Autodesk Inventor part; units mm, degrees
(part 2 of 4)
  line L378 (5.5115, 49.3393) -> (5.5188, 49.3267)
  arc A125 (6.0858, 49.2107) -> (6.0188, 49.4607) centre (5.5858, 49.2107) ccw
  arc A126 (5.4445, 49.5893) -> (5.5115, 49.3393) centre (5.9445, 49.5893) ccw
  arc A127 (5.9445, 49.7233) -> (6.0115, 49.4733) centre (6.4445, 49.7233) ccw
  arc A128 (4.8374, 49.2618) -> (4.7704, 49.5118) centre (4.3374, 49.2618) ccw
  line L379 (4.2751, 50.3697) -> (4.7704, 49.5118)
  line L380 (4.8128, 49.4383) -> (3.7356, 50.3041) construction
  line L381 (6.0188, 49.4607) -> (6.0115, 49.4733)
  arc A129 (2.9678, 49.0767) -> (2.9008, 49.3267) centre (2.4678, 49.0767) ccw
  arc A130 (3.4678, 49.2107) -> (3.4008, 49.4607) centre (2.9678, 49.2107) ccw
  arc A131 (6.0858, 42.4055) -> (6.1549, 42.1519) centre (6.5858, 42.4055) ccw
  line L382 (6.0858, 42.4055) -> (6.0858, 49.2107)
  line L383 (5.5858, 49.0767) -> (5.5858, 42.2693)
  line L384 (6.0858, 49.2776) -> (5.5858, 42.2012) construction
  line L385 (6.0858, 42.2012) -> (5.5858, 49.2776) construction
  arc A132 (5.5858, 42.2693) -> (5.6549, 42.0157) centre (6.0858, 42.2693) ccw
  line L386 (6.0513, 42.328) -> (9.5345, 35.4232) construction
  line L387 (5.6549, 42.0157) -> (9.4309, 35.5993)
  line L388 (9.9655, 35.6768) -> (5.6203, 42.0744) construction
  line L389 (9.9309, 35.7355) -> (6.1549, 42.1519)
  arc A133 (9.5, 35.3457) -> (9.4309, 35.5993) centre (9, 35.3457) ccw
  arc A134 (10, 35.4819) -> (9.9309, 35.7355) centre (9.5, 35.4819) ccw
  line L390 (9.5, 35.3457) -> (9.5, 34.85)
  line L391 (9.5, 34.85) -> (8.35, 34.85)
  line L392 (8.35, 34.85) -> (8.35, 34.05)
  line L393 (10, 34.85) -> (9.5, 35.55) construction
  line L394 (10, 35.55) -> (9.5, 34.85) construction
  line L395 (10, 34.85) -> (10, 35.4819)
  line L396 (8.35, 34.05) -> (11.15, 34.05)
  line L397 (9.5, 34.85) -> (10, 34.85)
  line L398 (11.15, 34.85) -> (10, 34.85)
  line L399 (11.15, 34.05) -> (11.15, 34.85)
  line L400 (8.35, 14.55) -> (11.15, 14.55)
  line L401 (8.35, 15.35) -> (8.35, 14.55)
  line L402 (9.5, 15.35) -> (8.35, 15.35)
  line L403 (9.5, 15.35) -> (10, 15.35)
  line L404 (11.15, 14.55) -> (11.15, 15.35)
  line L405 (11.15, 15.35) -> (10, 15.35)
  line L406 (9.5, 15.8491) -> (9.5, 15.35)
  line L407 (10, 15.35) -> (10, 15.983)
  line L408 (9.75, 15.35) -> (9.75, 16.05)
  line L409 (10, 15.35) -> (9.5, 16.05) construction
  line L410 (10, 16.05) -> (9.5, 15.35) construction
  line L411 (10, 16.05) -> (9.5, 16.05)
  arc A135 (9.5, 15.8491) -> (9.4331, 16.099) centre (9, 15.8491) ccw
  line L412 (9.5335, 15.9251) -> (9.9665, 16.1749)
  arc A136 (10, 15.983) -> (9.9331, 16.2329) centre (9.5, 15.983) ccw
  arc A137 (10, -3.517) -> (9.933, -3.267) centre (9.5, -3.517) ccw
  line L413 (9.5335, -3.575) -> (9.9665, -3.325)
  line L414 (9.933, -3.267) -> (3.5348, 7.8151)
  line L415 (9.9665, -3.325) -> (3.0013, 7.7391) construction
  line L416 (3.0348, 7.6811) -> (9.433, -3.401)
  line L417 (3.4343, 7.9891) -> (9.5335, -3.575) construction
  arc A138 (3.4678, 8.0651) -> (3.5348, 7.8151) centre (3.9678, 8.0651) ccw
  arc A139 (2.9678, 7.9311) -> (3.0348, 7.6811) centre (3.4678, 7.9311) ccw
  arc A140 (9.5, -3.651) -> (9.433, -3.401) centre (9, -3.651) ccw
  line L418 (10, -3.45) -> (9.5, -3.45)
  line L419 (9.5, -3.651) -> (9.5, -4.15)
  line L420 (10, -4.15) -> (10, -3.517)
  line L421 (9.5, -4.15) -> (8.35, -4.15)
  line L422 (9.5, -4.15) -> (10, -4.15)
  line L423 (11.15, -4.15) -> (10, -4.15)
  line L424 (8.35, -4.15) -> (8.35, -4.95)
  line L425 (8.35, -4.95) -> (11.15, -4.95)
  line L426 (11.15, -4.95) -> (11.15, -4.15)
  arc A141 (2.1588, -9.1677) -> (2.2258, -9.4177) centre (2.6588, -9.1677) ccw
  arc A142 (1.6588, -9.3016) -> (1.7258, -9.5516) centre (2.1588, -9.3016) ccw
  line L427 (0.3498, -26.5344) -> (0.3498, 49.0767)
  line L428 (0.8498, 49.2107) -> (0.8498, -26.4004)
  line L429 (1.6588, 49.0767) -> (1.6588, -9.3016)
  line L430 (2.1588, 49.2776) -> (1.6588, -9.3686) construction
  line L431 (2.1588, -9.3686) -> (1.6588, 49.2776) construction
  line L432 (2.1588, -9.1677) -> (2.1588, 49.2107)
  line L433 (2.9678, 7.9311) -> (2.9678, 49.0767)
  line L434 (3.4678, 7.8641) -> (2.9678, 49.2776) construction
  line L435 (3.4678, 49.2776) -> (2.9678, 7.8641) construction
  line L436 (3.4678, 49.2107) -> (3.4678, 8.0651)
  line L437 (4.3374, 49.1278) -> (4.3374, 25.0639)
  line L438 (4.8374, 25.1978) -> (4.8374, 49.2618)
  line L439 (4.8374, 49.3098) -> (4.3374, 25.002) construction
  line L440 (4.8374, 25.002) -> (4.3374, 49.3098) construction
  line L441 (9.5335, -23.075) -> (9.9665, -22.825)
  line L442 (1.7258, -9.5516) -> (9.433, -22.901)
  line L443 (2.1253, -9.2436) -> (9.5335, -23.075) construction
  line L444 (9.9665, -22.825) -> (1.6923, -9.4936) construction
  line L445 (2.1253, -9.2436) -> (1.6923, -9.4936)
  line L446 (9.933, -22.767) -> (2.2258, -9.4177)
  line L447 (9.5, -23.65) -> (10, -23.65)
  line L448 (9.5, -23.151) -> (9.5, -23.65)
  line L449 (10, -23.65) -> (10, -23.017)
  line L450 (10, -23.65) -> (9.5, -22.95) construction
  line L451 (10, -22.95) -> (9.5, -22.95)
  line L452 (10, -22.95) -> (9.5, -23.65) construction
  arc A143 (9.5, -23.151) -> (9.433, -22.901) centre (9, -23.151) ccw
  line L453 (8.35, -24.45) -> (11.15, -24.45)
  arc A144 (10, -23.017) -> (9.933, -22.767) centre (9.5, -23.017) ccw
  line L454 (11.15, -23.65) -> (10, -23.65)
  line L455 (11.15, -24.45) -> (11.15, -23.65)
  arc A145 (0.8498, -26.4004) -> (0.9168, -26.6504) centre (1.3498, -26.4004) ccw
  line L456 (9.5, -23.65) -> (8.35, -23.65)
  line L457 (8.35, -23.65) -> (8.35, -24.45)
  line L458 (9.933, -42.267) -> (0.9168, -26.6504)
  line L459 (9.9665, -42.325) -> (0.3833, -26.7264) construction
  line L460 (0.8163, -26.4764) -> (9.5335, -42.575) construction
  line L461 (0.4168, -26.7844) -> (9.433, -42.401)
  arc A146 (0.3498, -26.5344) -> (0.4168, -26.7844) centre (0.8498, -26.5344) ccw
  line L462 (0.8163, -26.4764) -> (0.3833, -26.7264)
  line L463 (9.75, -48.75) -> (9.75, -43.95)
  line L464 (11.15, -43.95) -> (8.35, -43.95)
  line L465 (11.15, -43.15) -> (11.15, -43.95)
  arc A147 (9.5, -42.651) -> (9.433, -42.401) centre (9, -42.651) ccw
  arc A148 (10, -42.517) -> (9.933, -42.267) centre (9.5, -42.517) ccw
  line L466 (9.5, -42.651) -> (9.5, -43.15)
  line L467 (8.35, -43.15) -> (9.5, -43.15)
  line L468 (8.35, -43.95) -> (8.35, -43.15)
  line L469 (10, -43.15) -> (10, -42.517)
  line L470 (10, -42.45) -> (9.5, -43.15) construction
  line L471 (9.5, -43.15) -> (10, -43.15)
  line L472 (10, -43.15) -> (11.15, -43.15)
  line L473 (10, -43.15) -> (9.5, -42.45) construction
  line L474 (9.9331, 16.2329) -> (4.9043, 24.9479)
  line L475 (9.9665, 16.1749) -> (4.3679, 24.8771) construction
  line L476 (4.801, 25.127) -> (9.5335, 15.9251) construction
  line L477 (4.4043, 24.814) -> (9.4331, 16.099)
  arc A149 (4.8374, 25.1978) -> (4.9043, 24.9479) centre (5.3374, 25.1978) ccw
  arc A150 (4.3374, 25.0639) -> (4.4043, 24.814) centre (4.8374, 25.0639) ccw
  line L478 (-11.15, 54.35) -> (-11.15, 53.55)
  line L479 (-10.0555, 54.35) -> (-11.15, 54.35)
  line L480 (-11.15, 53.55) -> (-8.35, 53.55)
  line L481 (-8.35, 54.35) -> (-9.5705, 54.35)
  line L482 (-8.35, 53.55) -> (-8.35, 54.35)
  line L483 (-10.0555, 54.35) -> (-10.0555, 60.0191)
  line L484 (-10.0555, 60.0191) -> (-9.5705, 60.0191)
  line L485 (-9.5705, 60.0191) -> (-9.5705, 54.35)
  line L486 (-9.5705, 60.0191) -> (-10.0168, 54.35) construction
  line L487 (-9.5705, 54.2285) -> (-10.0555, 60.0191) construction
  line L488 (-9.5705, 54.35) -> (-10.0555, 54.35)
  circle A151 centre (-9.8055, 60.0191) radius 0.75
  line L489 (-22.0555, 60.0187) -> (-21.5555, 60.0187)
  circle A152 centre (-21.8055, 60.0191) radius 0.75
  line L490 (-17.5555, 60.0191) -> (-18.0555, 60.0191)
  circle A153 centre (-17.8055, 60.0191) radius 0.75
  line L491 (-13.5555, 60.0191) -> (-14.0555, 60.0191)
  circle A154 centre (-13.8055, 60.0191) radius 0.75
  arc A155 (-19.2919, 52.8573) -> (-19.2249, 52.6073) centre (-18.7919, 52.8573) ccw
  arc A156 (-19.7919, 52.7233) -> (-19.7249, 52.4733) centre (-19.2919, 52.7233) ccw
  line L492 (-19.2919, 55.5191) -> (-19.2919, 52.8573)
  line L493 (-19.2919, 55.5191) -> (-19.7919, 52.6564) construction
  line L494 (-19.2919, 52.6564) -> (-19.7919, 55.5191) construction
  line L495 (-19.7919, 55.5191) -> (-19.2919, 55.5191)
  circle A157 centre (-19.5419, 55.5191) radius 0.75
  line L496 (-17.5555, 60.0191) -> (-18.0555, 51.916) construction
  line L497 (-17.5555, 51.916) -> (-18.0555, 60.0191) construction
  line L498 (-17.5555, 52.117) -> (-17.5555, 60.0191)
  line L499 (-18.0555, 60.0191) -> (-18.0555, 51.983)
  line L500 (-21.5555, 60.0187) -> (-21.5555, 54.5107)
  line L501 (-21.5555, 60.0187) -> (-22.0555, 54.3101) construction
  line L502 (-21.5555, 54.3101) -> (-22.0555, 60.0187) construction
  line L503 (-22.0555, 54.3767) -> (-22.0555, 60.0187)
  line L504 (-19.7919, 52.7233) -> (-19.7919, 55.5191)
  line L505 (-15.7919, 55.5191) -> (-15.2919, 55.5191)
  circle A158 centre (-15.5419, 55.5191) radius 0.75
  line L506 (-13.5555, 49.7233) -> (-13.5555, 60.0191)
  line L507 (-14.0555, 60.0191) -> (-13.5555, 49.5223) construction
  line L508 (-14.0555, 49.5223) -> (-13.5555, 60.0191) construction
  line L509 (-14.0555, 60.0191) -> (-14.0555, 49.5893)
  line L510 (-15.2919, 55.5191) -> (-15.2919, 50.6197)
  line L511 (-15.7919, 50.4857) -> (-15.7919, 55.5191)
  line L512 (-15.2919, 55.5191) -> (-15.7919, 50.4326) construction
  line L513 (-15.2919, 50.4326) -> (-15.7919, 55.5191) construction
  arc A159 (-15.7919, 50.4857) -> (-15.7249, 50.2357) centre (-15.2919, 50.4857) ccw
  arc A160 (-15.2919, 50.6197) -> (-15.2249, 50.3697) centre (-14.7919, 50.6197) ccw
  arc A161 (-21.5555, 54.5107) -> (-21.4885, 54.2607) centre (-21.0555, 54.5107) ccw
  arc A162 (-22.0555, 54.3767) -> (-21.9885, 54.1267) centre (-21.5555, 54.3767) ccw
  arc A163 (-19.1502, 49.0767) -> (-19.2172, 49.3267) centre (-19.6502, 49.0767) ccw
  line L514 (-21.589, 54.4347) -> (-19.1167, 49.1526) construction
  line L515 (-21.4885, 54.2607) -> (-18.7172, 49.4607)
  line L516 (-19.2172, 49.3267) -> (-21.9885, 54.1267)
  line L517 (-18.6837, 49.4026) -> (-22.022, 54.1847) construction
  arc A164 (-17.3412, 49.2107) -> (-17.4082, 49.4607) centre (-17.8412, 49.2107) ccw
  arc A165 (-17.8412, 49.0767) -> (-17.9082, 49.3267) centre (-18.3412, 49.0767) ccw
  arc A166 (-18.6502, 49.2107) -> (-18.7172, 49.4607) centre (-19.1502, 49.2107) ccw
  line L518 (-16.0992, 49.4607) -> (-17.4885, 51.867)
  line L519 (-16.0657, 49.4026) -> (-18.022, 51.791) construction
  line L520 (-17.589, 52.041) -> (-16.4987, 49.1526) construction
  line L521 (-17.9885, 51.733) -> (-16.5992, 49.3267)
  line L522 (-19.3254, 52.7814) -> (-17.8077, 49.1526) construction
  line L523 (-19.2249, 52.6073) -> (-17.4082, 49.4607)
  line L524 (-17.9082, 49.3267) -> (-19.7249, 52.4733)
  line L525 (-17.3747, 49.4026) -> (-19.7584, 52.5314) construction
  arc A167 (-17.5555, 52.117) -> (-17.4885, 51.867) centre (-17.0555, 52.117) ccw
  arc A168 (-18.0555, 51.983) -> (-17.9885, 51.733) centre (-17.5555, 51.983) ccw
  line L526 (-15.2296, 49.3778) -> (-15.7249, 50.2357)
  line L527 (-15.3314, 50.5541) -> (-15.1202, 49.1883) construction
  arc A169 (-15.1626, 49.1278) -> (-15.2296, 49.3778) centre (-15.6626, 49.1278) ccw
  arc A170 (-13.9142, 49.0767) -> (-13.9812, 49.3267) centre (-14.4142, 49.0767) ccw
  line L528 (-13.9885, 49.3393) -> (-13.9812, 49.3267)
  arc A171 (-13.4142, 49.2107) -> (-13.4812, 49.4607) centre (-13.9142, 49.2107) ccw
  arc A172 (-14.0555, 49.5893) -> (-13.9885, 49.3393) centre (-13.5555, 49.5893) ccw
  arc A173 (-13.5555, 49.7233) -> (-13.4885, 49.4733) centre (-13.0555, 49.7233) ccw
  arc A174 (-14.6626, 49.2618) -> (-14.7296, 49.5118) centre (-15.1626, 49.2618) ccw
  line L529 (-15.2249, 50.3697) -> (-14.7296, 49.5118)
  line L530 (-14.6872, 49.4383) -> (-15.7644, 50.3041) construction
  line L531 (-13.4812, 49.4607) -> (-13.4885, 49.4733)
  arc A175 (-16.5322, 49.0767) -> (-16.5992, 49.3267) centre (-17.0322, 49.0767) ccw
  arc A176 (-16.0322, 49.2107) -> (-16.0992, 49.4607) centre (-16.5322, 49.2107) ccw
  arc A177 (-13.4142, 42.4055) -> (-13.3451, 42.1519) centre (-12.9142, 42.4055) ccw
  line L532 (-13.4142, 42.4055) -> (-13.4142, 49.2107)
  line L533 (-13.9142, 49.0767) -> (-13.9142, 42.2693)
  line L534 (-13.4142, 49.2776) -> (-13.9142, 42.2012) construction
  line L535 (-13.4142, 42.2012) -> (-13.9142, 49.2776) construction
  arc A178 (-13.9142, 42.2693) -> (-13.8451, 42.0157) centre (-13.4142, 42.2693) ccw
  line L536 (-13.4487, 42.328) -> (-9.9655, 35.4232) construction
  line L537 (-13.8451, 42.0157) -> (-10.0691, 35.5993)
  line L538 (-9.5345, 35.6768) -> (-13.8797, 42.0744) construction
  line L539 (-9.5691, 35.7355) -> (-13.3451, 42.1519)
  arc A179 (-10, 35.3457) -> (-10.0691, 35.5993) centre (-10.5, 35.3457) ccw
  arc A180 (-9.5, 35.4819) -> (-9.5691, 35.7355) centre (-10, 35.4819) ccw
  line L540 (-10, 35.3457) -> (-10, 34.85)
  line L541 (-10, 34.85) -> (-11.15, 34.85)
  line L542 (-11.15, 34.85) -> (-11.15, 34.05)
  line L543 (-9.5, 34.85) -> (-10, 35.55) construction
  line L544 (-9.5, 35.55) -> (-10, 34.85) construction
  line L545 (-9.5, 34.85) -> (-9.5, 35.4819)
  line L546 (-11.15, 34.05) -> (-8.35, 34.05)
  line L547 (-10, 34.85) -> (-9.5, 34.85)
  line L548 (-8.35, 34.85) -> (-9.5, 34.85)
  line L549 (-8.35, 34.05) -> (-8.35, 34.85)
  line L550 (-11.15, 14.55) -> (-8.35, 14.55)
  line L551 (-11.15, 15.35) -> (-11.15, 14.55)
  line L552 (-10, 15.35) -> (-11.15, 15.35)
  line L553 (-10, 15.35) -> (-9.5, 15.35)
  line L554 (-8.35, 14.55) -> (-8.35, 15.35)
  line L555 (-8.35, 15.35) -> (-9.5, 15.35)
  line L556 (-10, 15.8491) -> (-10, 15.35)
  line L557 (-9.5, 15.35) -> (-9.5, 15.983)
  line L558 (-9.75, 15.35) -> (-9.75, 16.05)
  line L559 (-9.5, 15.35) -> (-10, 16.05) construction
  line L560 (-9.5, 16.05) -> (-10, 15.35) construction
  line L561 (-9.5, 16.05) -> (-10, 16.05)
  arc A181 (-10, 15.8491) -> (-10.0669, 16.099) centre (-10.5, 15.8491) ccw
  line L562 (-9.9665, 15.9251) -> (-9.5335, 16.1749)
  arc A182 (-9.5, 15.983) -> (-9.5669, 16.2329) centre (-10, 15.983) ccw
  arc A183 (-9.5, -3.517) -> (-9.567, -3.267) centre (-10, -3.517) ccw
  line L563 (-9.9665, -3.575) -> (-9.5335, -3.325)
  line L564 (-9.567, -3.267) -> (-15.9652, 7.8151)
  line L565 (-9.5335, -3.325) -> (-16.4987, 7.7391) construction
  line L566 (-16.4652, 7.6811) -> (-10.067, -3.401)
  line L567 (-16.0657, 7.9891) -> (-9.9665, -3.575) construction
  arc A184 (-16.0322, 8.0651) -> (-15.9652, 7.8151) centre (-15.5322, 8.0651) ccw
  arc A185 (-16.5322, 7.9311) -> (-16.4652, 7.6811) centre (-16.0322, 7.9311) ccw
  arc A186 (-10, -3.651) -> (-10.067, -3.401) centre (-10.5, -3.651) ccw
  line L568 (-9.5, -3.45) -> (-10, -3.45)
  line L569 (-10, -3.651) -> (-10, -4.15)
  line L570 (-9.5, -4.15) -> (-9.5, -3.517)
  line L571 (-10, -4.15) -> (-11.15, -4.15)
  line L572 (-10, -4.15) -> (-9.5, -4.15)
  line L573 (-8.35, -4.15) -> (-9.5, -4.15)
  line L574 (-11.15, -4.15) -> (-11.15, -4.95)
  line L575 (-11.15, -4.95) -> (-8.35, -4.95)
  line L576 (-8.35, -4.95) -> (-8.35, -4.15)
  arc A187 (-17.3412, -9.1677) -> (-17.2742, -9.4177) centre (-16.8412, -9.1677) ccw
  arc A188 (-17.8412, -9.3016) -> (-17.7742, -9.5516) centre (-17.3412, -9.3016) ccw
  line L577 (-19.1502, -26.5344) -> (-19.1502, 49.0767)
  line L578 (-18.6502, 49.2107) -> (-18.6502, -26.4004)
  line L579 (-17.8412, 49.0767) -> (-17.8412, -9.3016)
  line L580 (-17.3412, 49.2776) -> (-17.8412, -9.3686) construction
  line L581 (-17.3412, -9.3686) -> (-17.8412, 49.2776) construction
  line L582 (-17.3412, -9.1677) -> (-17.3412, 49.2107)
  line L583 (-16.5322, 7.9311) -> (-16.5322, 49.0767)
  line L584 (-16.0322, 7.8641) -> (-16.5322, 49.2776) construction
  line L585 (-16.0322, 49.2776) -> (-16.5322, 7.8641) construction
  line L586 (-16.0322, 49.2107) -> (-16.0322, 8.0651)
  line L587 (-15.1626, 49.1278) -> (-15.1626, 25.0639)
  line L588 (-14.6626, 25.1978) -> (-14.6626, 49.2618)
  line L589 (-14.6626, 49.3098) -> (-15.1626, 25.002) construction
  line L590 (-14.6626, 25.002) -> (-15.1626, 49.3098) construction
  line L591 (-9.9665, -23.075) -> (-9.5335, -22.825)
  line L592 (-17.7742, -9.5516) -> (-10.067, -22.901)
  line L593 (-17.3747, -9.2436) -> (-9.9665, -23.075) construction
  line L594 (-9.5335, -22.825) -> (-17.8077, -9.4936) construction
  line L595 (-17.3747, -9.2436) -> (-17.8077, -9.4936)
  line L596 (-9.567, -22.767) -> (-17.2742, -9.4177)
  line L597 (-10, -23.65) -> (-9.5, -23.65)
  line L598 (-10, -23.151) -> (-10, -23.65)
  line L599 (-9.5, -23.65) -> (-9.5, -23.017)
  line L600 (-9.5, -23.65) -> (-10, -22.95) construction
  line L601 (-9.5, -22.95) -> (-10, -22.95)
  line L602 (-9.5, -22.95) -> (-10, -23.65) construction
  arc A189 (-10, -23.151) -> (-10.067, -22.901) centre (-10.5, -23.151) ccw
  line L603 (-11.15, -24.45) -> (-8.35, -24.45)
  arc A190 (-9.5, -23.017) -> (-9.567, -22.767) centre (-10, -23.017) ccw
  line L604 (-8.35, -23.65) -> (-9.5, -23.65)
  line L605 (-8.35, -24.45) -> (-8.35, -23.65)
  arc A191 (-18.6502, -26.4004) -> (-18.5832, -26.6504) centre (-18.1502, -26.4004) ccw
  line L606 (-10, -23.65) -> (-11.15, -23.65)
  line L607 (-11.15, -23.65) -> (-11.15, -24.45)
  line L608 (-9.567, -42.267) -> (-18.5832, -26.6504)
  line L609 (-9.5335, -42.325) -> (-19.1167, -26.7264) construction
  line L610 (-18.6837, -26.4764) -> (-9.9665, -42.575) construction
  line L611 (-19.0832, -26.7844) -> (-10.067, -42.401)
  arc A192 (-19.1502, -26.5344) -> (-19.0832, -26.7844) centre (-18.6502, -26.5344) ccw
  line L612 (-18.6837, -26.4764) -> (-19.1167, -26.7264)
  line L613 (-9.75, -48.75) -> (-9.75, -43.95)
  line L614 (-8.35, -43.95) -> (-11.15, -43.95)
  line L615 (-8.35, -43.15) -> (-8.35, -43.95)
  arc A193 (-10, -42.651) -> (-10.067, -42.401) centre (-10.5, -42.651) ccw
  arc A194 (-9.5, -42.517) -> (-9.567, -42.267) centre (-10, -42.517) ccw
  line L616 (-10, -42.651) -> (-10, -43.15)
  line L617 (-11.15, -43.15) -> (-10, -43.15)
  line L618 (-11.15, -43.95) -> (-11.15, -43.15)
  line L619 (-9.5, -43.15) -> (-9.5, -42.517)
  line L620 (-9.5, -42.45) -> (-10, -43.15) construction
  line L621 (-10, -43.15) -> (-9.5, -43.15)
  line L622 (-9.5, -43.15) -> (-8.35, -43.15)
  line L623 (-9.5, -43.15) -> (-10, -42.45) construction
  line L624 (-9.5669, 16.2329) -> (-14.5957, 24.9479)
  line L625 (-9.5335, 16.1749) -> (-15.1321, 24.8771) construction
  line L626 (-14.699, 25.127) -> (-9.9665, 15.9251) construction
  line L627 (-15.0957, 24.814) -> (-10.0669, 16.099)
  arc A195 (-14.6626, 25.1978) -> (-14.5957, 24.9479) centre (-14.1626, 25.1978) ccw
  arc A196 (-15.1626, 25.0639) -> (-15.0957, 24.814) centre (-14.6626, 25.0639) ccw
  line L628 (-30.65, 54.35) -> (-30.65, 53.55)
  line L629 (-29.5555, 54.35) -> (-30.65, 54.35)
  line L630 (-30.65, 53.55) -> (-27.85, 53.55)
  line L631 (-27.85, 54.35) -> (-29.0705, 54.35)
  line L632 (-27.85, 53.55) -> (-27.85, 54.35)
  line L633 (-29.5555, 54.35) -> (-29.5555, 60.0191)
  line L634 (-29.5555, 60.0191) -> (-29.0705, 60.0191)
  line L635 (-29.0705, 60.0191) -> (-29.0705, 54.35)
  line L636 (-29.0705, 60.0191) -> (-29.5168, 54.35) construction
  line L637 (-29.0705, 54.2285) -> (-29.5555, 60.0191) construction
  line L638 (-29.0705, 54.35) -> (-29.5555, 54.35)
  circle A197 centre (-29.3055, 60.0191) radius 0.75
  line L639 (-41.5555, 60.0187) -> (-41.0555, 60.0187)
  circle A198 centre (-41.3055, 60.0191) radius 0.75
  line L640 (-37.0555, 60.0191) -> (-37.5555, 60.0191)
  circle A199 centre (-37.3055, 60.0191) radius 0.75
  line L641 (-33.0555, 60.0191) -> (-33.5555, 60.0191)
  circle A200 centre (-33.3055, 60.0191) radius 0.75
  arc A201 (-38.7919, 52.8573) -> (-38.7249, 52.6073) centre (-38.2919, 52.8573) ccw
  arc A202 (-39.2919, 52.7233) -> (-39.2249, 52.4733) centre (-38.7919, 52.7233) ccw
  line L642 (-38.7919, 55.5191) -> (-38.7919, 52.8573)
  line L643 (-38.7919, 55.5191) -> (-39.2919, 52.6564) construction
  line L644 (-38.7919, 52.6564) -> (-39.2919, 55.5191) construction
  line L645 (-39.2919, 55.5191) -> (-38.7919, 55.5191)
  circle A203 centre (-39.0419, 55.5191) radius 0.75
  line L646 (-37.0555, 60.0191) -> (-37.5555, 51.916) construction
  line L647 (-37.0555, 51.916) -> (-37.5555, 60.0191) construction
  line L648 (-37.0555, 52.117) -> (-37.0555, 60.0191)
  line L649 (-37.5555, 60.0191) -> (-37.5555, 51.983)
  line L650 (-41.0555, 60.0187) -> (-41.0555, 54.5107)
  line L651 (-41.0555, 60.0187) -> (-41.5555, 54.3101) construction
  line L652 (-41.0555, 54.3101) -> (-41.5555, 60.0187) construction
  line L653 (-41.5555, 54.3767) -> (-41.5555, 60.0187)
  line L654 (-39.2919, 52.7233) -> (-39.2919, 55.5191)
  line L655 (-35.2919, 55.5191) -> (-34.7919, 55.5191)
  circle A204 centre (-35.0419, 55.5191) radius 0.75
  line L656 (-33.0555, 49.7233) -> (-33.0555, 60.0191)
  line L657 (-33.5555, 60.0191) -> (-33.0555, 49.5223) construction
  line L658 (-33.5555, 49.5223) -> (-33.0555, 60.0191) construction
  line L659 (-33.5555, 60.0191) -> (-33.5555, 49.5893)
  line L660 (-34.7919, 55.5191) -> (-34.7919, 50.6197)
  line L661 (-35.2919, 50.4857) -> (-35.2919, 55.5191)
  line L662 (-34.7919, 55.5191) -> (-35.2919, 50.4326) construction
  line L663 (-34.7919, 50.4326) -> (-35.2919, 55.5191) construction
  arc A205 (-35.2919, 50.4857) -> (-35.2249, 50.2357) centre (-34.7919, 50.4857) ccw
  arc A206 (-34.7919, 50.6197) -> (-34.7249, 50.3697) centre (-34.2919, 50.6197) ccw
  arc A207 (-41.0555, 54.5107) -> (-40.9885, 54.2607) centre (-40.5555, 54.5107) ccw
  arc A208 (-41.5555, 54.3767) -> (-41.4885, 54.1267) centre (-41.0555, 54.3767) ccw
  arc A209 (-38.6502, 49.0767) -> (-38.7172, 49.3267) centre (-39.1502, 49.0767) ccw
  line L664 (-41.089, 54.4347) -> (-38.6167, 49.1526) construction
  line L665 (-40.9885, 54.2607) -> (-38.2172, 49.4607)
  line L666 (-38.7172, 49.3267) -> (-41.4885, 54.1267)
  line L667 (-38.1837, 49.4026) -> (-41.522, 54.1847) construction
  arc A210 (-36.8412, 49.2107) -> (-36.9082, 49.4607) centre (-37.3412, 49.2107) ccw
  arc A211 (-37.3412, 49.0767) -> (-37.4082, 49.3267) centre (-37.8412, 49.0767) ccw
  arc A212 (-38.1502, 49.2107) -> (-38.2172, 49.4607) centre (-38.6502, 49.2107) ccw
  line L668 (-35.5992, 49.4607) -> (-36.9885, 51.867)
  line L669 (-35.5657, 49.4026) -> (-37.522, 51.791) construction
  line L670 (-37.089, 52.041) -> (-35.9987, 49.1526) construction
  line L671 (-37.4885, 51.733) -> (-36.0992, 49.3267)
  line L672 (-38.8254, 52.7814) -> (-37.3077, 49.1526) construction
  line L673 (-38.7249, 52.6073) -> (-36.9082, 49.4607)
  line L674 (-37.4082, 49.3267) -> (-39.2249, 52.4733)
  line L675 (-36.8747, 49.4026) -> (-39.2584, 52.5314) construction
  arc A213 (-37.0555, 52.117) -> (-36.9885, 51.867) centre (-36.5555, 52.117) ccw
  arc A214 (-37.5555, 51.983) -> (-37.4885, 51.733) centre (-37.0555, 51.983) ccw
  line L676 (-34.7296, 49.3778) -> (-35.2249, 50.2357)
  line L677 (-34.8314, 50.5541) -> (-34.6202, 49.1883) construction
  arc A215 (-34.6626, 49.1278) -> (-34.7296, 49.3778) centre (-35.1626, 49.1278) ccw
  arc A216 (-33.4142, 49.0767) -> (-33.4812, 49.3267) centre (-33.9142, 49.0767) ccw
  line L678 (-33.4885, 49.3393) -> (-33.4812, 49.3267)
  arc A217 (-32.9142, 49.2107) -> (-32.9812, 49.4607) centre (-33.4142, 49.2107) ccw
  arc A218 (-33.5555, 49.5893) -> (-33.4885, 49.3393) centre (-33.0555, 49.5893) ccw
  arc A219 (-33.0555, 49.7233) -> (-32.9885, 49.4733) centre (-32.5555, 49.7233) ccw
  arc A220 (-34.1626, 49.2618) -> (-34.2296, 49.5118) centre (-34.6626, 49.2618) ccw
  line L679 (-34.7249, 50.3697) -> (-34.2296, 49.5118)
  line L680 (-34.1872, 49.4383) -> (-35.2644, 50.3041) construction
  line L681 (-32.9812, 49.4607) -> (-32.9885, 49.4733)
  arc A221 (-36.0322, 49.0767) -> (-36.0992, 49.3267) centre (-36.5322, 49.0767) ccw
  arc A222 (-35.5322, 49.2107) -> (-35.5992, 49.4607) centre (-36.0322, 49.2107) ccw
  arc A223 (-32.9142, 42.4055) -> (-32.8451, 42.1519) centre (-32.4142, 42.4055) ccw
  line L682 (-32.9142, 42.4055) -> (-32.9142, 49.2107)
  line L683 (-33.4142, 49.0767) -> (-33.4142, 42.2693)
  line L684 (-32.9142, 49.2776) -> (-33.4142, 42.2012) construction
  line L685 (-32.9142, 42.2012) -> (-33.4142, 49.2776) construction
  arc A224 (-33.4142, 42.2693) -> (-33.3451, 42.0157) centre (-32.9142, 42.2693) ccw
  line L686 (-32.9487, 42.328) -> (-29.4655, 35.4232) construction
  line L687 (-33.3451, 42.0157) -> (-29.5691, 35.5993)
  line L688 (-29.0345, 35.6768) -> (-33.3797, 42.0744) construction
  line L689 (-29.0691, 35.7355) -> (-32.8451, 42.1519)
  arc A225 (-29.5, 35.3457) -> (-29.5691, 35.5993) centre (-30, 35.3457) ccw
  arc A226 (-29, 35.4819) -> (-29.0691, 35.7355) centre (-29.5, 35.4819) ccw
  line L690 (-29.5, 35.3457) -> (-29.5, 34.85)
  line L691 (-29.5, 34.85) -> (-30.65, 34.85)
  line L692 (-30.65, 34.85) -> (-30.65, 34.05)
  line L693 (-29, 34.85) -> (-29.5, 35.55) construction
  line L694 (-29, 35.55) -> (-29.5, 34.85) construction
  line L695 (-29, 34.85) -> (-29, 35.4819)
  line L696 (-30.65, 34.05) -> (-27.85, 34.05)
  line L697 (-29.5, 34.85) -> (-29, 34.85)
  line L698 (-27.85, 34.85) -> (-29, 34.85)
  line L699 (-27.85, 34.05) -> (-27.85, 34.85)
  line L700 (-30.65, 14.55) -> (-27.85, 14.55)
  line L701 (-30.65, 15.35) -> (-30.65, 14.55)
  line L702 (-29.5, 15.35) -> (-30.65, 15.35)
  line L703 (-29.5, 15.35) -> (-29, 15.35)
  line L704 (-27.85, 14.55) -> (-27.85, 15.35)
  line L705 (-27.85, 15.35) -> (-29, 15.35)
  line L706 (-29.5, 15.8491) -> (-29.5, 15.35)
  line L707 (-29, 15.35) -> (-29, 15.983)
  line L708 (-29.25, 15.35) -> (-29.25, 16.05)
  line L709 (-29, 15.35) -> (-29.5, 16.05) construction
  line L710 (-29, 16.05) -> (-29.5, 15.35) construction
  line L711 (-29, 16.05) -> (-29.5, 16.05)
  arc A227 (-29.5, 15.8491) -> (-29.5669, 16.099) centre (-30, 15.8491) ccw
  line L712 (-29.4665, 15.9251) -> (-29.0335, 16.1749)
  arc A228 (-29, 15.983) -> (-29.0669, 16.2329) centre (-29.5, 15.983) ccw
  arc A229 (-29, -3.517) -> (-29.067, -3.267) centre (-29.5, -3.517) ccw
  line L713 (-29.4665, -3.575) -> (-29.0335, -3.325)
  line L714 (-29.067, -3.267) -> (-35.4652, 7.8151)
  line L715 (-29.0335, -3.325) -> (-35.9987, 7.7391) construction
  line L716 (-35.9652, 7.6811) -> (-29.567, -3.401)
  line L717 (-35.5657, 7.9891) -> (-29.4665, -3.575) construction
  arc A230 (-35.5322, 8.0651) -> (-35.4652, 7.8151) centre (-35.0322, 8.0651) ccw
  arc A231 (-36.0322, 7.9311) -> (-35.9652, 7.6811) centre (-35.5322, 7.9311) ccw
  arc A232 (-29.5, -3.651) -> (-29.567, -3.401) centre (-30, -3.651) ccw
  line L718 (-29, -3.45) -> (-29.5, -3.45)
  line L719 (-29.5, -3.651) -> (-29.5, -4.15)
  line L720 (-29, -4.15) -> (-29, -3.517)
  line L721 (-29.5, -4.15) -> (-30.65, -4.15)
  line L722 (-29.5, -4.15) -> (-29, -4.15)
  line L723 (-27.85, -4.15) -> (-29, -4.15)
  line L724 (-30.65, -4.15) -> (-30.65, -4.95)
  line L725 (-30.65, -4.95) -> (-27.85, -4.95)
  line L726 (-27.85, -4.95) -> (-27.85, -4.15)
  arc A233 (-36.8412, -9.1677) -> (-36.7742, -9.4177) centre (-36.3412, -9.1677) ccw
  arc A234 (-37.3412, -9.3016) -> (-37.2742, -9.5516) centre (-36.8412, -9.3016) ccw
  line L727 (-38.6502, -26.5344) -> (-38.6502, 49.0767)
  line L728 (-38.1502, 49.2107) -> (-38.1502, -26.4004)
  line L729 (-37.3412, 49.0767) -> (-37.3412, -9.3016)
  line L730 (-36.8412, 49.2776) -> (-37.3412, -9.3686) construction
  line L731 (-36.8412, -9.3686) -> (-37.3412, 49.2776) construction
  line L732 (-36.8412, -9.1677) -> (-36.8412, 49.2107)
  line L733 (-36.0322, 7.9311) -> (-36.0322, 49.0767)
  line L734 (-35.5322, 7.8641) -> (-36.0322, 49.2776) construction
  line L735 (-35.5322, 49.2776) -> (-36.0322, 7.8641) construction
  line L736 (-35.5322, 49.2107) -> (-35.5322, 8.0651)
  line L737 (-34.6626, 49.1278) -> (-34.6626, 25.0639)
  line L738 (-34.1626, 25.1978) -> (-34.1626, 49.2618)
  line L739 (-34.1626, 49.3098) -> (-34.6626, 25.002) construction
  line L740 (-34.1626, 25.002) -> (-34.6626, 49.3098) construction
  line L741 (-29.4665, -23.075) -> (-29.0335, -22.825)
  line L742 (-37.2742, -9.5516) -> (-29.567, -22.901)
  line L743 (-36.8747, -9.2436) -> (-29.4665, -23.075) construction
  line L744 (-29.0335, -22.825) -> (-37.3077, -9.4936) construction
  line L745 (-36.8747, -9.2436) -> (-37.3077, -9.4936)
  line L746 (-29.067, -22.767) -> (-36.7742, -9.4177)
  line L747 (-29.5, -23.65) -> (-29, -23.65)
  line L748 (-29.5, -23.151) -> (-29.5, -23.65)
  line L749 (-29, -23.65) -> (-29, -23.017)
  line L750 (-29, -23.65) -> (-29.5, -22.95) construction
  line L751 (-29, -22.95) -> (-29.5, -22.95)
  line L752 (-29, -22.95) -> (-29.5, -23.65) construction
  arc A235 (-29.5, -23.151) -> (-29.567, -22.901) centre (-30, -23.151) ccw
  line L753 (-30.65, -24.45) -> (-27.85, -24.45)
  arc A236 (-29, -23.017) -> (-29.067, -22.767) centre (-29.5, -23.017) ccw
  line L754 (-27.85, -23.65) -> (-29, -23.65)
  line L755 (-27.85, -24.45) -> (-27.85, -23.65)
  arc A237 (-38.1502, -26.4004) -> (-38.0832, -26.6504) centre (-37.6502, -26.4004) ccw
  line L756 (-29.5, -23.65) -> (-30.65, -23.65)
  line L757 (-30.65, -23.65) -> (-30.65, -24.45)
  line L758 (-29.067, -42.267) -> (-38.0832, -26.6504)
  line L759 (-29.0335, -42.325) -> (-38.6167, -26.7264) construction
  line L760 (-38.1837, -26.4764) -> (-29.4665, -42.575) construction
  line L761 (-38.5832, -26.7844) -> (-29.567, -42.401)
  arc A238 (-38.6502, -26.5344) -> (-38.5832, -26.7844) centre (-38.1502, -26.5344) ccw
  line L762 (-38.1837, -26.4764) -> (-38.6167, -26.7264)
  line L763 (-29.25, -48.75) -> (-29.25, -43.95)
  line L764 (-27.85, -43.95) -> (-30.65, -43.95)
  line L765 (-27.85, -43.15) -> (-27.85, -43.95)
  arc A239 (-29.5, -42.651) -> (-29.567, -42.401) centre (-30, -42.651) ccw
  arc A240 (-29, -42.517) -> (-29.067, -42.267) centre (-29.5, -42.517) ccw
  line L766 (-29.5, -42.651) -> (-29.5, -43.15)
  line L767 (-30.65, -43.15) -> (-29.5, -43.15)
  line L768 (-30.65, -43.95) -> (-30.65, -43.15)
  line L769 (-29, -43.15) -> (-29, -42.517)
  line L770 (-29, -42.45) -> (-29.5, -43.15) construction
  line L771 (-29.5, -43.15) -> (-29, -43.15)
  line L772 (-29, -43.15) -> (-27.85, -43.15)
  line L773 (-29, -43.15) -> (-29.5, -42.45) construction
  line L774 (-29.0669, 16.2329) -> (-34.0957, 24.9479)
  line L775 (-29.0335, 16.1749) -> (-34.6321, 24.8771) construction
  line L776 (-34.199, 25.127) -> (-29.4665, 15.9251) construction
  line L777 (-34.5957, 24.814) -> (-29.5669, 16.099)
  arc A241 (-34.1626, 25.1978) -> (-34.0957, 24.9479) centre (-33.6626, 25.1978) ccw
  arc A242 (-34.6626, 25.0639) -> (-34.5957, 24.814) centre (-34.1626, 25.0639) ccw
  line L778 (19.2249, -52.6073) -> (17.4082, -49.4607)
  line L779 (15.7919, -50.4857) -> (15.7919, -55.5191)
  line L780 (15.2919, -55.5191) -> (15.2919, -50.6197)
  line L781 (15.2919, -55.5191) -> (15.7919, -50.4326) construction
  line L782 (15.2919, -50.4326) -> (15.7919, -55.5191) construction
  line L783 (16.0992, -49.4607) -> (17.4885, -51.867)
  line L784 (18.0555, -60.0191) -> (18.0555, -51.983)
  line L785 (17.5555, -51.916) -> (18.0555, -60.0191) construction
  line L786 (17.5555, -60.0191) -> (18.0555, -51.916) construction
  line L787 (17.5555, -52.117) -> (17.5555, -60.0191)
  line L788 (14.6872, -49.4383) -> (15.7644, -50.3041) construction
  line L789 (15.2249, -50.3697) -> (14.7296, -49.5118)
  line L790 (13.4812, -49.4607) -> (13.4885, -49.4733)
  line L791 (14.0555, -60.0191) -> (14.0555, -49.5893)
  line L792 (13.5555, -49.7233) -> (13.5555, -60.0191)
  line L793 (14.0555, -49.5223) -> (13.5555, -60.0191) construction
  line L794 (14.0555, -60.0191) -> (13.5555, -49.5223) construction
  line L795 (21.5555, -60.0187) -> (21.5555, -54.5107)
  line L796 (22.0555, -54.3767) -> (22.0555, -60.0187)
  line L797 (21.5555, -54.3101) -> (22.0555, -60.0187) construction
  line L798 (21.5555, -60.0187) -> (22.0555, -54.3101) construction
  line L799 (9.5705, -60.0191) -> (9.5705, -54.35)
  line L800 (10.0555, -60.0191) -> (9.5705, -60.0191)
  circle A243 centre (9.8055, -60.0191) radius 0.75
  line L801 (9.5705, -60.0191) -> (10.0168, -54.35) construction
  line L802 (9.5705, -54.35) -> (10.0555, -54.35)
  line L803 (10.0555, -54.35) -> (10.0555, -60.0191)
  line L804 (9.5705, -54.2285) -> (10.0555, -60.0191) construction
  arc A244 (14.0555, -49.5893) -> (13.9885, -49.3393) centre (13.5555, -49.5893) ccw
  arc A245 (14.6626, -49.2618) -> (14.7296, -49.5118) centre (15.1626, -49.2618) ccw
  arc A246 (13.9142, -49.0767) -> (13.9812, -49.3267) centre (14.4142, -49.0767) ccw
  arc A247 (13.5555, -49.7233) -> (13.4885, -49.4733) centre (13.0555, -49.7233) ccw
  arc A248 (13.4142, -49.2107) -> (13.4812, -49.4607) centre (13.9142, -49.2107) ccw
  line L805 (16.0657, -49.4026) -> (18.022, -51.791) construction
  line L806 (17.9885, -51.733) -> (16.5992, -49.3267)
  line L807 (17.589, -52.041) -> (16.4987, -49.1526) construction
  line L808 (21.4885, -54.2607) -> (18.7172, -49.4607)
  line L809 (16.0322, -49.2107) -> (16.0322, -8.0651)
  line L810 (16.0322, -49.2776) -> (16.5322, -7.8641) construction
  line L811 (16.0322, -7.8641) -> (16.5322, -49.2776) construction
  line L812 (16.5322, -7.9311) -> (16.5322, -49.0767)
  line L813 (17.3412, 9.1677) -> (17.3412, -49.2107)
  line L814 (17.8412, -49.0767) -> (17.8412, 9.3016)
  line L815 (17.3412, -49.2776) -> (17.8412, 9.3686) construction
  line L816 (18.6502, -49.2107) -> (18.6502, 26.4004)
  line L817 (19.1502, 26.5344) -> (19.1502, -49.0767)
  line L818 (17.3412, 9.3686) -> (17.8412, -49.2776) construction
  line L819 (17.3747, -49.4026) -> (19.7584, -52.5314) construction
  line L820 (18.6837, -49.4026) -> (22.022, -54.1847) construction
  line L821 (17.9082, -49.3267) -> (19.7249, -52.4733)
  line L822 (13.4142, -42.4055) -> (13.4142, -49.2107)
  line L823 (13.9142, -49.0767) -> (13.9142, -42.2693)
  line L824 (13.4142, -49.2776) -> (13.9142, -42.2012) construction
  line L825 (13.4142, -42.2012) -> (13.9142, -49.2776) construction
  line L826 (9.5691, -35.7355) -> (13.3451, -42.1519)
  line L827 (13.4487, -42.328) -> (9.9655, -35.4232) construction
  line L828 (13.8451, -42.0157) -> (10.0691, -35.5993)
  arc A249 (13.4142, -42.4055) -> (13.3451, -42.1519) centre (12.9142, -42.4055) ccw
  arc A250 (13.9142, -42.2693) -> (13.8451, -42.0157) centre (13.4142, -42.2693) ccw
  line L829 (9.5345, -35.6768) -> (13.8797, -42.0744) construction
  arc A251 (9.5, -35.4819) -> (9.5691, -35.7355) centre (10, -35.4819) ccw
  arc A252 (10, -35.3457) -> (10.0691, -35.5993) centre (10.5, -35.3457) ccw
  line L830 (10, -35.3457) -> (10, -34.85)
  line L831 (9.5, -35.55) -> (10, -34.85) construction
  line L832 (9.5, -34.85) -> (10, -35.55) construction
  line L833 (10, -34.85) -> (9.5, -34.85)
  line L834 (9.5, -34.85) -> (9.5, -35.4819)
  line L835 (13.9885, -49.3393) -> (13.9812, -49.3267)
  line L836 (14.6626, -25.1978) -> (14.6626, -49.2618)
  line L837 (15.1626, -49.1278) -> (15.1626, -25.0639)
  line L838 (14.6626, -25.002) -> (15.1626, -49.3098) construction
  line L839 (14.6626, -49.3098) -> (15.1626, -25.002) construction
  arc A253 (15.1626, -25.0639) -> (15.0957, -24.814) centre (14.6626, -25.0639) ccw
  arc A254 (14.6626, -25.1978) -> (14.5957, -24.9479) centre (14.1626, -25.1978) ccw
  line L840 (8.35, -34.85) -> (9.5, -34.85)
  line L841 (10, -34.85) -> (11.15, -34.85)
  line L842 (8.35, -34.05) -> (8.35, -34.85)
  line L843 (11.15, -34.05) -> (8.35, -34.05)
  line L844 (11.15, -34.85) -> (11.15, -34.05)
  arc A255 (9.5, -15.983) -> (9.5669, -16.2329) centre (10, -15.983) ccw
  line L845 (9.9665, -15.9251) -> (9.5335, -16.1749)
  line L846 (9.5669, -16.2329) -> (14.5957, -24.9479)
  line L847 (9.5335, -16.1749) -> (15.1321, -24.8771) construction
  line L848 (14.699, -25.127) -> (9.9665, -15.9251) construction
  line L849 (15.0957, -24.814) -> (10.0669, -16.099)
  line L850 (9.5, -16.05) -> (10, -16.05)
  arc A256 (10, -15.8491) -> (10.0669, -16.099) centre (10.5, -15.8491) ccw
  line L851 (9.75, -15.35) -> (9.75, -16.05)
  line L852 (9.5, -15.35) -> (10, -16.05) construction
  line L853 (9.5, -16.05) -> (10, -15.35) construction
  line L854 (10, -15.35) -> (9.5, -15.35)
  line L855 (8.35, -15.35) -> (9.5, -15.35)
  line L856 (11.15, -14.55) -> (8.35, -14.55)
  line L857 (8.35, -14.55) -> (8.35, -15.35)
  line L858 (9.5, -15.35) -> (9.5, -15.983)
  arc A257 (16.5322, -7.9311) -> (16.4652, -7.6811) centre (16.0322, -7.9311) ccw
  arc A258 (16.0322, -8.0651) -> (15.9652, -7.8151) centre (15.5322, -8.0651) ccw
  line L859 (10, -15.8491) -> (10, -15.35)
  line L860 (10, -15.35) -> (11.15, -15.35)
  line L861 (11.15, -15.35) -> (11.15, -14.55)
  line L862 (9.567, 3.267) -> (15.9652, -7.8151)
  line L863 (16.4652, -7.6811) -> (10.067, 3.401)
  line L864 (9.9665, 3.575) -> (9.5335, 3.325)
  line L865 (9.5335, 3.325) -> (16.4987, -7.7391) construction
  line L866 (16.0657, -7.9891) -> (9.9665, 3.575) construction
  line L867 (9.5, 3.45) -> (10, 3.45)
  arc A259 (9.5, 3.517) -> (9.567, 3.267) centre (10, 3.517) ccw
  line L868 (11.15, 4.15) -> (11.15, 4.95)
  line L869 (10, 4.15) -> (11.15, 4.15)
  line L870 (10, 3.651) -> (10, 4.15)
  line L871 (10, 4.15) -> (9.5, 4.15)
  arc A260 (10, 3.651) -> (10.067, 3.401) centre (10.5, 3.651) ccw
  line L872 (9.5, 4.15) -> (9.5, 3.517)
  line L873 (11.15, 4.95) -> (8.35, 4.95)
  line L874 (8.35, 4.95) -> (8.35, 4.15)
  line L875 (8.35, 4.15) -> (9.5, 4.15)
  line L876 (17.3747, 9.2436) -> (17.8077, 9.4936)
  arc A261 (17.3412, 9.1677) -> (17.2742, 9.4177) centre (16.8412, 9.1677) ccw
  arc A262 (17.8412, 9.3016) -> (17.7742, 9.5516) centre (17.3412, 9.3016) ccw
  line L877 (9.567, 42.267) -> (18.5832, 26.6504)
  line L878 (18.6837, 26.4764) -> (19.1167, 26.7264)
  line L879 (19.0832, 26.7844) -> (10.067, 42.401)
  line L880 (9.5335, 42.325) -> (19.1167, 26.7264) construction
  line L881 (18.6837, 26.4764) -> (9.9665, 42.575) construction
  arc A263 (19.1502, 26.5344) -> (19.0832, 26.7844) centre (18.6502, 26.5344) ccw
  arc A264 (18.6502, 26.4004) -> (18.5832, 26.6504) centre (18.1502, 26.4004) ccw
  line L882 (10, 23.65) -> (11.15, 23.65)
  line L883 (11.15, 23.65) -> (11.15, 24.45)
  line L884 (8.35, 24.45) -> (8.35, 23.65)
  line L885 (8.35, 23.65) -> (9.5, 23.65)
  line L886 (11.15, 24.45) -> (8.35, 24.45)
  line L887 (8.35, 43.95) -> (11.15, 43.95)
  line L888 (10, 42.651) -> (10, 43.15)
  line L889 (9.5, 43.15) -> (9.5, 42.517)
  line L890 (9.5, 43.15) -> (10, 42.45) construction
  line L891 (9.5, 42.45) -> (10, 43.15) construction
  arc A265 (10, 42.651) -> (10.067, 42.401) centre (10.5, 42.651) ccw
  arc A266 (9.5, 42.517) -> (9.567, 42.267) centre (10, 42.517) ccw
  line L892 (11.15, 43.95) -> (11.15, 43.15)
  line L893 (11.15, 43.15) -> (10, 43.15)
  line L894 (10, 43.15) -> (9.5, 43.15)
  line L895 (9.75, 48.75) -> (9.75, 43.95)
  line L896 (9.5, 43.15) -> (8.35, 43.15)
  line L897 (8.35, 43.15) -> (8.35, 43.95)
  line L898 (9.567, 22.767) -> (17.2742, 9.4177)
  line L899 (17.7742, 9.5516) -> (10.067, 22.901)
  line L900 (9.9665, 23.075) -> (9.5335, 22.825)
  line L901 (9.5335, 22.825) -> (17.8077, 9.4936) construction
  line L902 (17.3747, 9.2436) -> (9.9665, 23.075) construction
  line L903 (10, 23.65) -> (9.5, 23.65)
  line L904 (10, 23.151) -> (10, 23.65)
  line L905 (9.5, 23.65) -> (9.5, 23.017)
  line L906 (9.5, 23.65) -> (10, 22.95) construction
  line L907 (9.5, 22.95) -> (10, 23.65) construction
  line L908 (9.5, 22.95) -> (10, 22.95)
  arc A267 (10, 23.151) -> (10.067, 22.901) centre (10.5, 23.151) ccw
  arc A268 (9.5, 23.017) -> (9.567, 22.767) centre (10, 23.017) ccw
  line L909 (19.2172, -49.3267) -> (21.9885, -54.1267)
  line L910 (19.2919, -55.5191) -> (19.7919, -52.6564) construction
  line L911 (19.2919, -52.6564) -> (19.7919, -55.5191) construction
  line L912 (19.7919, -52.7233) -> (19.7919, -55.5191)
  circle A269 centre (19.5419, -55.5191) radius 0.75
  line L913 (19.2919, -55.5191) -> (19.2919, -52.8573)
  arc A270 (17.5555, -52.117) -> (17.4885, -51.867) centre (17.0555, -52.117) ccw
  arc A271 (18.0555, -51.983) -> (17.9885, -51.733) centre (17.5555, -51.983) ccw
  arc A272 (19.2919, -52.8573) -> (19.2249, -52.6073) centre (18.7919, -52.8573) ccw
  arc A273 (19.7919, -52.7233) -> (19.7249, -52.4733) centre (19.2919, -52.7233) ccw
  line L914 (21.589, -54.4347) -> (19.1167, -49.1526) construction
  arc A274 (19.1502, -49.0767) -> (19.2172, -49.3267) centre (19.6502, -49.0767) ccw
  arc A275 (18.6502, -49.2107) -> (18.7172, -49.4607) centre (19.1502, -49.2107) ccw
  arc A276 (17.3412, -49.2107) -> (17.4082, -49.4607) centre (17.8412, -49.2107) ccw
  arc A277 (17.8412, -49.0767) -> (17.9082, -49.3267) centre (18.3412, -49.0767) ccw
  line L915 (19.3254, -52.7814) -> (17.8077, -49.1526) construction
  line L916 (22.0555, -60.0187) -> (21.5555, -60.0187)
  circle A278 centre (21.8055, -60.0191) radius 0.75
  line L917 (19.7919, -55.5191) -> (19.2919, -55.5191)
  line L918 (15.2296, -49.3778) -> (15.7249, -50.2357)
  line L919 (15.3314, -50.5541) -> (15.1202, -49.1883) construction
  arc A279 (15.1626, -49.1278) -> (15.2296, -49.3778) centre (15.6626, -49.1278) ccw
  arc A280 (15.7919, -50.4857) -> (15.7249, -50.2357) centre (15.2919, -50.4857) ccw
  arc A281 (16.0322, -49.2107) -> (16.0992, -49.4607) centre (16.5322, -49.2107) ccw
  arc A282 (16.5322, -49.0767) -> (16.5992, -49.3267) centre (17.0322, -49.0767) ccw
  arc A283 (15.2919, -50.6197) -> (15.2249, -50.3697) centre (14.7919, -50.6197) ccw
  arc A284 (22.0555, -54.3767) -> (21.9885, -54.1267) centre (21.5555, -54.3767) ccw
  arc A285 (21.5555, -54.5107) -> (21.4885, -54.2607) centre (21.0555, -54.5107) ccw
  line L920 (15.7919, -55.5191) -> (15.2919, -55.5191)
  circle A286 centre (15.5419, -55.5191) radius 0.75
  line L921 (17.5555, -60.0191) -> (18.0555, -60.0191)
  circle A287 centre (17.8055, -60.0191) radius 0.75
  line L922 (13.5555, -60.0191) -> (14.0555, -60.0191)
  circle A288 centre (13.8055, -60.0191) radius 0.75
  line L923 (11.15, -53.55) -> (8.35, -53.55)
  line L924 (10.0555, -54.35) -> (11.15, -54.35)
  line L925 (11.15, -54.35) -> (11.15, -53.55)
  line L926 (8.35, -54.35) -> (9.5705, -54.35)
  line L927 (8.35, -53.55) -> (8.35, -54.35)
  line L928 (-0.2751, -52.6073) -> (-2.0918, -49.4607)
  line L929 (-3.7081, -50.4857) -> (-3.7081, -55.5191)
  line L930 (-4.2081, -55.5191) -> (-4.2081, -50.6197)
  line L931 (-4.2081, -55.5191) -> (-3.7081, -50.4326) construction
  line L932 (-4.2081, -50.4326) -> (-3.7081, -55.5191) construction
  line L933 (-3.4008, -49.4607) -> (-2.0115, -51.867)
  line L934 (-1.4445, -60.0191) -> (-1.4445, -51.983)
  line L935 (-1.9445, -51.916) -> (-1.4445, -60.0191) construction
  line L936 (-1.9445, -60.0191) -> (-1.4445, -51.916) construction
  line L937 (-1.9445, -52.117) -> (-1.9445, -60.0191)
  line L938 (-4.8128, -49.4383) -> (-3.7356, -50.3041) construction
  line L939 (-4.2751, -50.3697) -> (-4.7704, -49.5118)
  line L940 (-6.0188, -49.4607) -> (-6.0115, -49.4733)
  line L941 (-5.4445, -60.0191) -> (-5.4445, -49.5893)
  line L942 (-5.9445, -49.7233) -> (-5.9445, -60.0191)
  line L943 (-5.4445, -49.5223) -> (-5.9445, -60.0191) construction
  line L944 (-5.4445, -60.0191) -> (-5.9445, -49.5223) construction
  line L945 (2.0555, -60.0187) -> (2.0555, -54.5107)
  line L946 (2.5555, -54.3767) -> (2.5555, -60.0187)
  line L947 (2.0555, -54.3101) -> (2.5555, -60.0187) construction
  line L948 (2.0555, -60.0187) -> (2.5555, -54.3101) construction
  line L949 (-9.9295, -60.0191) -> (-9.9295, -54.35)
  line L950 (-9.4445, -60.0191) -> (-9.9295, -60.0191)
  circle A289 centre (-9.6945, -60.0191) radius 0.75
  line L951 (-9.9295, -60.0191) -> (-9.4832, -54.35) construction
  line L952 (-9.9295, -54.35) -> (-9.4445, -54.35)
  line L953 (-9.4445, -54.35) -> (-9.4445, -60.0191)
  line L954 (-9.9295, -54.2285) -> (-9.4445, -60.0191) construction
  arc A290 (-5.4445, -49.5893) -> (-5.5115, -49.3393) centre (-5.9445, -49.5893) ccw
  arc A291 (-4.8374, -49.2618) -> (-4.7704, -49.5118) centre (-4.3374, -49.2618) ccw
  arc A292 (-5.5858, -49.0767) -> (-5.5188, -49.3267) centre (-5.0858, -49.0767) ccw
  arc A293 (-5.9445, -49.7233) -> (-6.0115, -49.4733) centre (-6.4445, -49.7233) ccw
  arc A294 (-6.0858, -49.2107) -> (-6.0188, -49.4607) centre (-5.5858, -49.2107) ccw
  line L955 (-3.4343, -49.4026) -> (-1.478, -51.791) construction
  line L956 (-1.5115, -51.733) -> (-2.9008, -49.3267)
  line L957 (-1.911, -52.041) -> (-3.0013, -49.1526) construction
  line L958 (1.9885, -54.2607) -> (-0.7828, -49.4607)
  line L959 (-3.4678, -49.2107) -> (-3.4678, -8.0651)
  line L960 (-3.4678, -49.2776) -> (-2.9678, -7.8641) construction
  line L961 (-3.4678, -7.8641) -> (-2.9678, -49.2776) construction
  line L962 (-2.9678, -7.9311) -> (-2.9678, -49.0767)
  line L963 (-2.1588, 9.1677) -> (-2.1588, -49.2107)
  line L964 (-1.6588, -49.0767) -> (-1.6588, 9.3016)
  line L965 (-2.1588, -49.2776) -> (-1.6588, 9.3686) construction
  line L966 (-0.8498, -49.2107) -> (-0.8498, 26.4004)
  line L967 (-0.3498, 26.5344) -> (-0.3498, -49.0767)
  line L968 (-2.1588, 9.3686) -> (-1.6588, -49.2776) construction
  line L969 (-2.1253, -49.4026) -> (0.2584, -52.5314) construction
  line L970 (-0.8163, -49.4026) -> (2.522, -54.1847) construction
  line L971 (-1.5918, -49.3267) -> (0.2249, -52.4733)
  line L972 (-6.0858, -42.4055) -> (-6.0858, -49.2107)
  line L973 (-5.5858, -49.0767) -> (-5.5858, -42.2693)
  line L974 (-6.0858, -49.2776) -> (-5.5858, -42.2012) construction
  line L975 (-6.0858, -42.2012) -> (-5.5858, -49.2776) construction
  line L976 (-9.9309, -35.7355) -> (-6.1549, -42.1519)
  line L977 (-6.0513, -42.328) -> (-9.5345, -35.4232) construction
  line L978 (-5.6549, -42.0157) -> (-9.4309, -35.5993)
  arc A295 (-6.0858, -42.4055) -> (-6.1549, -42.1519) centre (-6.5858, -42.4055) ccw
  arc A296 (-5.5858, -42.2693) -> (-5.6549, -42.0157) centre (-6.0858, -42.2693) ccw
  line L979 (-9.9655, -35.6768) -> (-5.6203, -42.0744) construction
  arc A297 (-10, -35.4819) -> (-9.9309, -35.7355) centre (-9.5, -35.4819) ccw
  arc A298 (-9.5, -35.3457) -> (-9.4309, -35.5993) centre (-9, -35.3457) ccw
  line L980 (-9.5, -35.3457) -> (-9.5, -34.85)
  line L981 (-10, -35.55) -> (-9.5, -34.85) construction
  line L982 (-10, -34.85) -> (-9.5, -35.55) construction
  line L983 (-9.5, -34.85) -> (-10, -34.85)
  line L984 (-10, -34.85) -> (-10, -35.4819)
  line L985 (-5.5115, -49.3393) -> (-5.5188, -49.3267)
  line L986 (-4.8374, -25.1978) -> (-4.8374, -49.2618)
  line L987 (-4.3374, -49.1278) -> (-4.3374, -25.0639)
  line L988 (-4.8374, -25.002) -> (-4.3374, -49.3098) construction
  line L989 (-4.8374, -49.3098) -> (-4.3374, -25.002) construction
  arc A299 (-4.3374, -25.0639) -> (-4.4043, -24.814) centre (-4.8374, -25.0639) ccw
  arc A300 (-4.8374, -25.1978) -> (-4.9043, -24.9479) centre (-5.3374, -25.1978) ccw
  line L990 (-11.15, -34.85) -> (-10, -34.85)
  line L991 (-9.5, -34.85) -> (-8.35, -34.85)
  line L992 (-11.15, -34.05) -> (-11.15, -34.85)
  line L993 (-8.35, -34.05) -> (-11.15, -34.05)
  line L994 (-8.35, -34.85) -> (-8.35, -34.05)
  arc A301 (-10, -15.983) -> (-9.9331, -16.2329) centre (-9.5, -15.983) ccw
  line L995 (-9.5335, -15.9251) -> (-9.9665, -16.1749)
  line L996 (-9.9331, -16.2329) -> (-4.9043, -24.9479)
  line L997 (-9.9665, -16.1749) -> (-4.3679, -24.8771) construction
  line L998 (-4.801, -25.127) -> (-9.5335, -15.9251) construction
  line L999 (-4.4043, -24.814) -> (-9.4331, -16.099)
  line L1000 (-10, -16.05) -> (-9.5, -16.05)
  arc A302 (-9.5, -15.8491) -> (-9.4331, -16.099) centre (-9, -15.8491) ccw
  line L1001 (-9.75, -15.35) -> (-9.75, -16.05)
  line L1002 (-10, -15.35) -> (-9.5, -16.05) construction
  line L1003 (-10, -16.05) -> (-9.5, -15.35) construction
  line L1004 (-9.5, -15.35) -> (-10, -15.35)
  line L1005 (-11.15, -15.35) -> (-10, -15.35)
  line L1006 (-8.35, -14.55) -> (-11.15, -14.55)
  line L1007 (-11.15, -14.55) -> (-11.15, -15.35)
  line L1008 (-10, -15.35) -> (-10, -15.983)
  arc A303 (-2.9678, -7.9311) -> (-3.0348, -7.6811) centre (-3.4678, -7.9311) ccw
  arc A304 (-3.4678, -8.0651) -> (-3.5348, -7.8151) centre (-3.9678, -8.0651) ccw
  line L1009 (-9.5, -15.8491) -> (-9.5, -15.35)
  line L1010 (-9.5, -15.35) -> (-8.35, -15.35)
  line L1011 (-8.35, -15.35) -> (-8.35, -14.55)
  line L1012 (-9.933, 3.267) -> (-3.5348, -7.8151)
  line L1013 (-3.0348, -7.6811) -> (-9.433, 3.401)
  line L1014 (-9.5335, 3.575) -> (-9.9665, 3.325)
  line L1015 (-9.9665, 3.325) -> (-3.0013, -7.7391) construction
  line L1016 (-3.4343, -7.9891) -> (-9.5335, 3.575) construction
  line L1017 (-10, 3.45) -> (-9.5, 3.45)
  arc A305 (-10, 3.517) -> (-9.933, 3.267) centre (-9.5, 3.517) ccw
  line L1018 (-8.35, 4.15) -> (-8.35, 4.95)
  line L1019 (-9.5, 4.15) -> (-8.35, 4.15)
  line L1020 (-9.5, 3.651) -> (-9.5, 4.15)
  line L1021 (-9.5, 4.15) -> (-10, 4.15)
  arc A306 (-9.5, 3.651) -> (-9.433, 3.401) centre (-9, 3.651) ccw
  line L1022 (-10, 4.15) -> (-10, 3.517)
  line L1023 (-8.35, 4.95) -> (-11.15, 4.95)
  line L1024 (-11.15, 4.95) -> (-11.15, 4.15)
  line L1025 (-11.15, 4.15) -> (-10, 4.15)
  line L1026 (-2.1253, 9.2436) -> (-1.6923, 9.4936)
  arc A307 (-2.1588, 9.1677) -> (-2.2258, 9.4177) centre (-2.6588, 9.1677) ccw
  arc A308 (-1.6588, 9.3016) -> (-1.7258, 9.5516) centre (-2.1588, 9.3016) ccw
  line L1027 (-9.933, 42.267) -> (-0.9168, 26.6504)
  line L1028 (-0.8163, 26.4764) -> (-0.3833, 26.7264)
  line L1029 (-0.4168, 26.7844) -> (-9.433, 42.401)
  line L1030 (-9.9665, 42.325) -> (-0.3833, 26.7264) construction
  line L1031 (-0.8163, 26.4764) -> (-9.5335, 42.575) construction
  arc A309 (-0.3498, 26.5344) -> (-0.4168, 26.7844) centre (-0.8498, 26.5344) ccw
  arc A310 (-0.8498, 26.4004) -> (-0.9168, 26.6504) centre (-1.3498, 26.4004) ccw
  line L1032 (-9.5, 23.65) -> (-8.35, 23.65)
  line L1033 (-8.35, 23.65) -> (-8.35, 24.45)
  line L1034 (-11.15, 24.45) -> (-11.15, 23.65)
  line L1035 (-11.15, 23.65) -> (-10, 23.65)